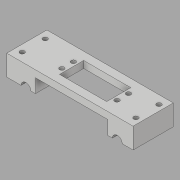
# Autodesk Inventor part: g_servo mount 1
Saved by Autodesk Inventor 2019 (Build 230136000, 136)
## iProperties
Created: 2021-10-30
Part Number: g_servo mount 1
Material: Generic
Document SubType Name: Modeling
Designer: Mohamed
Density: 1 g/cm^3
Appearance: Default
Author: Mohamed
Autodesk Inventor part; units mm, degrees
ref_plane "YZ Plane" through (0, 0, 0) normal (1, 0, 0) x (0, 1, 0)
ref_plane "XZ Plane" through (0, 0, 0) normal (0, 1, 0) x (-1, 0, 0)
ref_plane "XY Plane" through (0, 0, 0) normal (0, 0, 1) x (1, 0, 0)
sketch "Sketch1" plane through (0, 0, 0) normal (0, 1, 0) x (-1, 0, 0)
  line L0 (0, 0) -> (0, -35)
  line L1 (0, -35) -> (110, -35)
  line L2 (110, -35) -> (110, 0)
  line L3 (110, 0) -> (0, 0)
  line L4 (0, -35) -> (30, -35)
  line L5 (30, -17.5) -> (30, -28)
  line L6 (30, -28) -> (30, -7)
  line L7 (30, -7) -> (71, -7)
  line L8 (71, -7) -> (71, -28)
  line L9 (71, -28) -> (30, -28)
  circle A0 centre (74.5, -12.5) radius 2
  circle A1 centre (74.5, -22.5) radius 2
  circle A2 centre (26.5, -22.5) radius 2
  circle A3 centre (26.5, -12.5) radius 2
  dimension "d0" = 35
  dimension "d1" = 110
  dimension "d4" = 21
  dimension "d5" = 41
  dimension "d6" = 21
  dimension "d10" = 4
  dimension "d11" = 4
  dimension "d15" = 4
  dimension "d16" = 4
  constraints: 20 end point, 5 perpendicular, 4 centre point, 2 point on line, 2 vertical
  measures "d0" distance of L0.start L0.end
  measures "d1" distance of L0.end L1.end
  measures "d4" distance of L5.end L6.end
  measures "d5" distance of L6.end L7.end
  measures "d6" distance of L7.end L8.end
  measures "d10" diameter of A0
  measures "d11" diameter of A1
  measures "d15" diameter of A2
  measures "d16" diameter of A3
extrude "Extrusion1" add sketch "Sketch1" along normal blind 6
sketch "Sketch2" plane through (0, 0, -35) normal (0, 0, -1) x (-1, 0, 0)
  line L0 (0, 0) -> (0, 6) projected
  line L1 (0, 0) -> (0, -12)
  line L2 (22, -12) -> (22, 0)
  line L3 (0, 0) -> (110, 0) projected
  line L4 (22, -12) -> (18, -12)
  arc A0 (18, -12) -> (9.5, -12) centre (13.75, -12) ccw
  line L5 (9.5, -12) -> (0, -12)
  line L6 (110, 0) -> (110, -12)
  line L7 (85, -12) -> (85, 0)
  arc A1 (97.5, -12) -> (89, -12) centre (93.25, -12) ccw
  line L8 (89, -12) -> (85, -12)
  line L9 (110, -12) -> (97.5, -12)
  dimension "d19" = 12
  dimension "d20" = 22
  dimension "d21" = 4
  dimension "d23" = 8.5
  dimension "d24" = 12
  dimension "d25" = 25
  dimension "d26" = 8.5
  dimension "d27" = 8.25
  constraints: 16 end point, 4 point on circle, 3 point on line, 2 centre point, 2 horizontal, 2 vertical, 1 perpendicular
  measures "d19" distance of L0.start L1.end
  measures "d20" distance of L1.end L2.start
  measures "d21" distance of L2.start L4.end
  measures "d23" diameter of A0
  measures "d24" distance of L3.end L6.end
  measures "d25" distance of L6.end L7.start
  measures "d26" diameter of A1
  measures "d27" distance of A1.centre L7.start
extrude "Extrusion2" add sketch "Sketch2" against normal blind 35
sketch "Sketch3" plane through (-110, -12, -35) normal (0, -1, 0) x (1, 0, 0)
  line L0 (0, 0) -> (0, 35) projected
  circle A0 centre (6, 7.5) radius 2
  circle A1 centre (6, 27.5) radius 2
  line L1 (110, 35) -> (110, 0) projected
  circle A2 centre (105, 27.5) radius 2
  circle A3 centre (105, 7.5) radius 2
  dimension "d33" = 4
  dimension "d34" = 4
  dimension "d38" = 4
  dimension "d39" = 4
  constraints: 4 centre point
  measures "d33" diameter of A0
  measures "d34" diameter of A1
  measures "d38" diameter of A2
  measures "d39" diameter of A3
extrude "Extrusion3" cut sketch "Sketch3" against normal blind 18
body "Solid1"
